Autodesk Inventor part; units mm, degrees
(part 5 of 13)
  line L1582 (2.4, 58.0134) -> (2.4, 59.1669)
  arc A1584 (2.4, 59.1669) -> (2.274, 59.1669) centre (2.337, 59.1669) ccw
  line L1583 (2.274, 59.1669) -> (2.274, 58.0134)
  arc A1585 (2.274, 58.0134) -> (2.4, 58.0134) centre (2.337, 58.0134) ccw
  line L1584 (2.337, 59.2299) -> (2.1578, 59.2299)
  arc A1586 (2.1578, 59.2299) -> (2.1578, 59.1039) centre (2.1578, 59.1669) ccw
  line L1585 (2.1578, 59.1039) -> (2.337, 59.1039)
  arc A1587 (2.337, 59.1039) -> (2.337, 59.2299) centre (2.337, 59.1669) ccw
  line L1586 (2.1337, 59.2251) -> (1.6865, 59.0398)
  arc A1588 (1.6865, 59.0398) -> (1.7347, 58.9234) centre (1.7106, 58.9816) ccw
  line L1587 (1.7347, 58.9234) -> (2.1819, 59.1087)
  arc A1589 (2.1819, 59.1087) -> (2.1337, 59.2251) centre (2.1578, 59.1669) ccw
  line L1588 (1.6661, 59.0261) -> (1.3238, 58.6838)
  arc A1590 (1.3238, 58.6838) -> (1.4128, 58.5948) centre (1.3683, 58.6393) ccw
  line L1589 (1.4128, 58.5948) -> (1.7551, 58.9371)
  arc A1591 (1.7551, 58.9371) -> (1.6661, 59.0261) centre (1.7106, 58.9816) ccw
  line L1590 (1.3101, 58.6634) -> (1.1248, 58.2162)
  arc A1592 (1.1248, 58.2162) -> (1.2412, 58.168) centre (1.183, 58.1921) ccw
  line L1591 (1.2412, 58.168) -> (1.4265, 58.6152)
  arc A1593 (1.4265, 58.6152) -> (1.3101, 58.6634) centre (1.3683, 58.6393) ccw
  line L1592 (1.12, 58.1921) -> (1.12, 58.0128)
  arc A1594 (1.12, 58.0128) -> (1.246, 58.0128) centre (1.183, 58.0128) ccw
  line L1593 (1.246, 58.0128) -> (1.246, 58.1921)
  arc A1595 (1.246, 58.1921) -> (1.12, 58.1921) centre (1.183, 58.1921) ccw
  line L1594 (1.183, 57.9498) -> (2.3365, 57.9498)
  arc A1596 (2.3365, 57.9498) -> (2.3365, 58.0758) centre (2.3365, 58.0128) ccw
  line L1595 (2.3365, 58.0758) -> (1.183, 58.0758)
  arc A1597 (1.183, 58.0758) -> (1.183, 57.9498) centre (1.183, 58.0128) ccw
  line L1596 (2.2735, 58.0128) -> (2.2735, 57.887)
  arc A1598 (2.2735, 57.887) -> (2.3995, 57.887) centre (2.3365, 57.887) ccw
  line L1597 (2.3995, 57.887) -> (2.3995, 58.0128)
  arc A1599 (2.3995, 58.0128) -> (2.2735, 58.0128) centre (2.3365, 58.0128) ccw
  line L1598 (2.3365, 57.95) -> (1.183, 57.95)
  arc A1600 (1.183, 57.95) -> (1.183, 57.824) centre (1.183, 57.887) ccw
  line L1599 (1.183, 57.824) -> (2.3365, 57.824)
  arc A1601 (2.3365, 57.824) -> (2.3365, 57.95) centre (2.3365, 57.887) ccw
  line L1600 (1.12, 57.887) -> (1.12, 57.7078)
  arc A1602 (1.12, 57.7078) -> (1.246, 57.7078) centre (1.183, 57.7078) ccw
  line L1601 (1.246, 57.7078) -> (1.246, 57.887)
  arc A1603 (1.246, 57.887) -> (1.12, 57.887) centre (1.183, 57.887) ccw
  line L1602 (1.1248, 57.6837) -> (1.3101, 57.2365)
  arc A1604 (1.3101, 57.2365) -> (1.4265, 57.2847) centre (1.3683, 57.2606) ccw
  line L1603 (1.4265, 57.2847) -> (1.2412, 57.7319)
  arc A1605 (1.2412, 57.7319) -> (1.1248, 57.6837) centre (1.183, 57.7078) ccw
  line L1604 (1.3238, 57.2161) -> (1.6661, 56.8738)
  arc A1606 (1.6661, 56.8738) -> (1.7551, 56.9628) centre (1.7106, 56.9183) ccw
  line L1605 (1.7551, 56.9628) -> (1.4128, 57.3051)
  arc A1607 (1.4128, 57.3051) -> (1.3238, 57.2161) centre (1.3683, 57.2606) ccw
  line L1606 (1.6865, 56.8601) -> (2.1337, 56.6748)
  arc A1608 (2.1337, 56.6748) -> (2.1819, 56.7912) centre (2.1578, 56.733) ccw
  line L1607 (2.1819, 56.7912) -> (1.7347, 56.9765)
  arc A1609 (1.7347, 56.9765) -> (1.6865, 56.8601) centre (1.7106, 56.9183) ccw
  line L1608 (3.5783, 54.2281) -> (3.5783, 54.6718)
  arc A1610 (3.5783, 54.6718) -> (3.4523, 54.6718) centre (3.5153, 54.6718) ccw
  line L1609 (3.4523, 54.6718) -> (3.4523, 54.2281)
  arc A1611 (3.4523, 54.2281) -> (3.5783, 54.2281) centre (3.5153, 54.2281) ccw
  line L1610 (3.5735, 54.6959) -> (3.4037, 55.1059)
  arc A1612 (3.4037, 55.1059) -> (3.2873, 55.0577) centre (3.3455, 55.0818) ccw
  line L1611 (3.2873, 55.0577) -> (3.4571, 54.6477)
  arc A1613 (3.4571, 54.6477) -> (3.5735, 54.6959) centre (3.5153, 54.6718) ccw
  line L1612 (3.39, 55.1263) -> (3.0763, 55.44)
  arc A1614 (3.0763, 55.44) -> (2.9873, 55.351) centre (3.0318, 55.3955) ccw
  line L1613 (2.9873, 55.351) -> (3.301, 55.0373)
  arc A1615 (3.301, 55.0373) -> (3.39, 55.1263) centre (3.3455, 55.0818) ccw
  line L1614 (3.0559, 55.4537) -> (2.6459, 55.6235)
  arc A1616 (2.6459, 55.6235) -> (2.5977, 55.5071) centre (2.6218, 55.5653) ccw
  line L1615 (2.5977, 55.5071) -> (3.0077, 55.3373)
  arc A1617 (3.0077, 55.3373) -> (3.0559, 55.4537) centre (3.0318, 55.3955) ccw
  line L1616 (2.6218, 55.6283) -> (2.1781, 55.6283)
  arc A1618 (2.1781, 55.6283) -> (2.1781, 55.5023) centre (2.1781, 55.5653) ccw
  line L1617 (2.1781, 55.5023) -> (2.6218, 55.5023)
  arc A1619 (2.6218, 55.5023) -> (2.6218, 55.6283) centre (2.6218, 55.5653) ccw
  line L1618 (2.154, 55.6235) -> (1.744, 55.4537)
  arc A1620 (1.744, 55.4537) -> (1.7922, 55.3373) centre (1.7681, 55.3955) ccw
  line L1619 (1.7922, 55.3373) -> (2.2022, 55.5071)
  arc A1621 (2.2022, 55.5071) -> (2.154, 55.6235) centre (2.1781, 55.5653) ccw
  line L1620 (1.7236, 55.44) -> (1.4099, 55.1263)
  arc A1622 (1.4099, 55.1263) -> (1.4989, 55.0373) centre (1.4544, 55.0818) ccw
  line L1621 (1.4989, 55.0373) -> (1.8126, 55.351)
  arc A1623 (1.8126, 55.351) -> (1.7236, 55.44) centre (1.7681, 55.3955) ccw
  line L1622 (1.3962, 55.1059) -> (1.2264, 54.6959)
  arc A1624 (1.2264, 54.6959) -> (1.3428, 54.6477) centre (1.2846, 54.6718) ccw
  line L1623 (1.3428, 54.6477) -> (1.5126, 55.0577)
  arc A1625 (1.5126, 55.0577) -> (1.3962, 55.1059) centre (1.4544, 55.0818) ccw
  line L1624 (1.2216, 54.6718) -> (1.2216, 54.2281)
  arc A1626 (1.2216, 54.2281) -> (1.3476, 54.2281) centre (1.2846, 54.2281) ccw
  line L1625 (1.3476, 54.2281) -> (1.3476, 54.6718)
  arc A1627 (1.3476, 54.6718) -> (1.2216, 54.6718) centre (1.2846, 54.6718) ccw
  line L1626 (1.2264, 54.204) -> (1.3962, 53.794)
  arc A1628 (1.3962, 53.794) -> (1.5126, 53.8422) centre (1.4544, 53.8181) ccw
  line L1627 (1.5126, 53.8422) -> (1.3428, 54.2522)
  arc A1629 (1.3428, 54.2522) -> (1.2264, 54.204) centre (1.2846, 54.2281) ccw
  line L1628 (1.4099, 53.7736) -> (1.7236, 53.4599)
  arc A1630 (1.7236, 53.4599) -> (1.8126, 53.5489) centre (1.7681, 53.5044) ccw
  line L1629 (1.8126, 53.5489) -> (1.4989, 53.8626)
  arc A1631 (1.4989, 53.8626) -> (1.4099, 53.7736) centre (1.4544, 53.8181) ccw
  line L1630 (1.744, 53.4462) -> (2.154, 53.2764)
  arc A1632 (2.154, 53.2764) -> (2.2022, 53.3928) centre (2.1781, 53.3346) ccw
  line L1631 (2.2022, 53.3928) -> (1.7922, 53.5626)
  arc A1633 (1.7922, 53.5626) -> (1.744, 53.4462) centre (1.7681, 53.5044) ccw
  line L1632 (2.1781, 53.2716) -> (2.6218, 53.2716)
  arc A1634 (2.6218, 53.2716) -> (2.6218, 53.3976) centre (2.6218, 53.3346) ccw
  line L1633 (2.6218, 53.3976) -> (2.1781, 53.3976)
  arc A1635 (2.1781, 53.3976) -> (2.1781, 53.2716) centre (2.1781, 53.3346) ccw
  line L1634 (2.6459, 53.2764) -> (3.0559, 53.4462)
  arc A1636 (3.0559, 53.4462) -> (3.0077, 53.5626) centre (3.0318, 53.5044) ccw
  line L1635 (3.0077, 53.5626) -> (2.5977, 53.3928)
  arc A1637 (2.5977, 53.3928) -> (2.6459, 53.2764) centre (2.6218, 53.3346) ccw
  line L1636 (3.0763, 53.4599) -> (3.39, 53.7736)
  arc A1638 (3.39, 53.7736) -> (3.301, 53.8626) centre (3.3455, 53.8181) ccw
  line L1637 (3.301, 53.8626) -> (2.9873, 53.5489)
  arc A1639 (2.9873, 53.5489) -> (3.0763, 53.4599) centre (3.0318, 53.5044) ccw
  line L1638 (3.4037, 53.794) -> (3.5735, 54.204)
  arc A1640 (3.5735, 54.204) -> (3.4571, 54.2522) centre (3.5153, 54.2281) ccw
  line L1639 (3.4571, 54.2522) -> (3.2873, 53.8422)
  arc A1641 (3.2873, 53.8422) -> (3.4037, 53.794) centre (3.3455, 53.8181) ccw
  line L1640 (2.1578, 42.67) -> (2.337, 42.67)
  arc A1642 (2.337, 42.67) -> (2.337, 42.796) centre (2.337, 42.733) ccw
  line L1641 (2.337, 42.796) -> (2.1578, 42.796)
  arc A1643 (2.1578, 42.796) -> (2.1578, 42.67) centre (2.1578, 42.733) ccw
  line L1642 (2.4, 42.733) -> (2.4, 43.8865)
  arc A1644 (2.4, 43.8865) -> (2.274, 43.8865) centre (2.337, 43.8865) ccw
  line L1643 (2.274, 43.8865) -> (2.274, 42.733)
  arc A1645 (2.274, 42.733) -> (2.4, 42.733) centre (2.337, 42.733) ccw
  line L1644 (2.337, 43.8235) -> (2.4628, 43.8235)
  arc A1646 (2.4628, 43.8235) -> (2.4628, 43.9495) centre (2.4628, 43.8865) ccw
  line L1645 (2.4628, 43.9495) -> (2.337, 43.9495)
  arc A1647 (2.337, 43.9495) -> (2.337, 43.8235) centre (2.337, 43.8865) ccw
  line L1646 (2.3998, 43.8865) -> (2.3998, 42.733)
  arc A1648 (2.3998, 42.733) -> (2.5258, 42.733) centre (2.4628, 42.733) ccw
  line L1647 (2.5258, 42.733) -> (2.5258, 43.8865)
  arc A1649 (2.5258, 43.8865) -> (2.3998, 43.8865) centre (2.4628, 43.8865) ccw
  line L1648 (2.4628, 42.67) -> (2.6421, 42.67)
  arc A1650 (2.6421, 42.67) -> (2.6421, 42.796) centre (2.6421, 42.733) ccw
  line L1649 (2.6421, 42.796) -> (2.4628, 42.796)
  arc A1651 (2.4628, 42.796) -> (2.4628, 42.67) centre (2.4628, 42.733) ccw
  line L1650 (2.6662, 42.6748) -> (3.1134, 42.8601)
  arc A1652 (3.1134, 42.8601) -> (3.0652, 42.9765) centre (3.0893, 42.9183) ccw
  line L1651 (3.0652, 42.9765) -> (2.618, 42.7912)
  arc A1653 (2.618, 42.7912) -> (2.6662, 42.6748) centre (2.6421, 42.733) ccw
  line L1652 (3.1338, 42.8738) -> (3.4761, 43.2161)
  arc A1654 (3.4761, 43.2161) -> (3.3871, 43.3051) centre (3.4316, 43.2606) ccw
  line L1653 (3.3871, 43.3051) -> (3.0448, 42.9628)
  arc A1655 (3.0448, 42.9628) -> (3.1338, 42.8738) centre (3.0893, 42.9183) ccw
  line L1654 (3.4898, 43.2365) -> (3.6751, 43.6837)
  arc A1656 (3.6751, 43.6837) -> (3.5587, 43.7319) centre (3.6169, 43.7078) ccw
  line L1655 (3.5587, 43.7319) -> (3.3734, 43.2847)
  arc A1657 (3.3734, 43.2847) -> (3.4898, 43.2365) centre (3.4316, 43.2606) ccw
  line L1656 (3.6799, 43.7078) -> (3.6799, 43.887)
  arc A1658 (3.6799, 43.887) -> (3.5539, 43.887) centre (3.6169, 43.887) ccw
  line L1657 (3.5539, 43.887) -> (3.5539, 43.7078)
  arc A1659 (3.5539, 43.7078) -> (3.6799, 43.7078) centre (3.6169, 43.7078) ccw
  line L1658 (3.6169, 43.95) -> (2.4634, 43.95)
  arc A1660 (2.4634, 43.95) -> (2.4634, 43.824) centre (2.4634, 43.887) ccw
  line L1659 (2.4634, 43.824) -> (3.6169, 43.824)
  arc A1661 (3.6169, 43.824) -> (3.6169, 43.95) centre (3.6169, 43.887) ccw
  line L1660 (2.5264, 43.887) -> (2.5264, 44.0128)
  arc A1662 (2.5264, 44.0128) -> (2.4004, 44.0128) centre (2.4634, 44.0128) ccw
  line L1661 (2.4004, 44.0128) -> (2.4004, 43.887)
  arc A1663 (2.4004, 43.887) -> (2.5264, 43.887) centre (2.4634, 43.887) ccw
  line L1662 (2.4634, 43.9498) -> (3.6169, 43.9498)
  arc A1664 (3.6169, 43.9498) -> (3.6169, 44.0758) centre (3.6169, 44.0128) ccw
  line L1663 (3.6169, 44.0758) -> (2.4634, 44.0758)
  arc A1665 (2.4634, 44.0758) -> (2.4634, 43.9498) centre (2.4634, 44.0128) ccw
  line L1664 (3.6799, 44.0128) -> (3.6799, 44.1921)
  arc A1666 (3.6799, 44.1921) -> (3.5539, 44.1921) centre (3.6169, 44.1921) ccw
  line L1665 (3.5539, 44.1921) -> (3.5539, 44.0128)
  arc A1667 (3.5539, 44.0128) -> (3.6799, 44.0128) centre (3.6169, 44.0128) ccw
  line L1666 (3.6751, 44.2162) -> (3.4898, 44.6634)
  arc A1668 (3.4898, 44.6634) -> (3.3734, 44.6152) centre (3.4316, 44.6393) ccw
  line L1667 (3.3734, 44.6152) -> (3.5587, 44.168)
  arc A1669 (3.5587, 44.168) -> (3.6751, 44.2162) centre (3.6169, 44.1921) ccw
  line L1668 (3.4761, 44.6838) -> (3.1338, 45.0261)
  arc A1670 (3.1338, 45.0261) -> (3.0448, 44.9371) centre (3.0893, 44.9816) ccw
  line L1669 (3.0448, 44.9371) -> (3.3871, 44.5948)
  arc A1671 (3.3871, 44.5948) -> (3.4761, 44.6838) centre (3.4316, 44.6393) ccw
  line L1670 (3.1134, 45.0398) -> (2.6662, 45.2251)
  arc A1672 (2.6662, 45.2251) -> (2.618, 45.1087) centre (2.6421, 45.1669) ccw
  line L1671 (2.618, 45.1087) -> (3.0652, 44.9234)
  arc A1673 (3.0652, 44.9234) -> (3.1134, 45.0398) centre (3.0893, 44.9816) ccw
  line L1672 (2.6421, 45.2299) -> (2.4628, 45.2299)
  arc A1674 (2.4628, 45.2299) -> (2.4628, 45.1039) centre (2.4628, 45.1669) ccw
  line L1673 (2.4628, 45.1039) -> (2.6421, 45.1039)
  arc A1675 (2.6421, 45.1039) -> (2.6421, 45.2299) centre (2.6421, 45.1669) ccw
  line L1674 (2.3998, 45.1669) -> (2.3998, 44.0134)
  arc A1676 (2.3998, 44.0134) -> (2.5258, 44.0134) centre (2.4628, 44.0134) ccw
  line L1675 (2.5258, 44.0134) -> (2.5258, 45.1669)
  arc A1677 (2.5258, 45.1669) -> (2.3998, 45.1669) centre (2.4628, 45.1669) ccw
  line L1676 (2.4628, 44.0764) -> (2.337, 44.0764)
  arc A1678 (2.337, 44.0764) -> (2.337, 43.9504) centre (2.337, 44.0134) ccw
  line L1677 (2.337, 43.9504) -> (2.4628, 43.9504)
  arc A1679 (2.4628, 43.9504) -> (2.4628, 44.0764) centre (2.4628, 44.0134) ccw
  line L1678 (2.4, 44.0134) -> (2.4, 45.1669)
  arc A1680 (2.4, 45.1669) -> (2.274, 45.1669) centre (2.337, 45.1669) ccw
  line L1679 (2.274, 45.1669) -> (2.274, 44.0134)
  arc A1681 (2.274, 44.0134) -> (2.4, 44.0134) centre (2.337, 44.0134) ccw
  line L1680 (2.337, 45.2299) -> (2.1578, 45.2299)
  arc A1682 (2.1578, 45.2299) -> (2.1578, 45.1039) centre (2.1578, 45.1669) ccw
  line L1681 (2.1578, 45.1039) -> (2.337, 45.1039)
  arc A1683 (2.337, 45.1039) -> (2.337, 45.2299) centre (2.337, 45.1669) ccw
  line L1682 (2.1337, 45.2251) -> (1.6865, 45.0398)
  arc A1684 (1.6865, 45.0398) -> (1.7347, 44.9234) centre (1.7106, 44.9816) ccw
  line L1683 (1.7347, 44.9234) -> (2.1819, 45.1087)
  arc A1685 (2.1819, 45.1087) -> (2.1337, 45.2251) centre (2.1578, 45.1669) ccw
  line L1684 (1.6661, 45.0261) -> (1.3238, 44.6838)
  arc A1686 (1.3238, 44.6838) -> (1.4128, 44.5948) centre (1.3683, 44.6393) ccw
  line L1685 (1.4128, 44.5948) -> (1.7551, 44.9371)
  arc A1687 (1.7551, 44.9371) -> (1.6661, 45.0261) centre (1.7106, 44.9816) ccw
  line L1686 (1.3101, 44.6634) -> (1.1248, 44.2162)
  arc A1688 (1.1248, 44.2162) -> (1.2412, 44.168) centre (1.183, 44.1921) ccw
  line L1687 (1.2412, 44.168) -> (1.4265, 44.6152)
  arc A1689 (1.4265, 44.6152) -> (1.3101, 44.6634) centre (1.3683, 44.6393) ccw
  line L1688 (1.12, 44.1921) -> (1.12, 44.0128)
  arc A1690 (1.12, 44.0128) -> (1.246, 44.0128) centre (1.183, 44.0128) ccw
  line L1689 (1.246, 44.0128) -> (1.246, 44.1921)
  arc A1691 (1.246, 44.1921) -> (1.12, 44.1921) centre (1.183, 44.1921) ccw
  line L1690 (1.183, 43.9498) -> (2.3365, 43.9498)
  arc A1692 (2.3365, 43.9498) -> (2.3365, 44.0758) centre (2.3365, 44.0128) ccw
  line L1691 (2.3365, 44.0758) -> (1.183, 44.0758)
  arc A1693 (1.183, 44.0758) -> (1.183, 43.9498) centre (1.183, 44.0128) ccw
  line L1692 (2.2735, 44.0128) -> (2.2735, 43.887)
  arc A1694 (2.2735, 43.887) -> (2.3995, 43.887) centre (2.3365, 43.887) ccw
  line L1693 (2.3995, 43.887) -> (2.3995, 44.0128)
  arc A1695 (2.3995, 44.0128) -> (2.2735, 44.0128) centre (2.3365, 44.0128) ccw
  line L1694 (2.3365, 43.95) -> (1.183, 43.95)
  arc A1696 (1.183, 43.95) -> (1.183, 43.824) centre (1.183, 43.887) ccw
  line L1695 (1.183, 43.824) -> (2.3365, 43.824)
  arc A1697 (2.3365, 43.824) -> (2.3365, 43.95) centre (2.3365, 43.887) ccw
  line L1696 (1.12, 43.887) -> (1.12, 43.7078)
  arc A1698 (1.12, 43.7078) -> (1.246, 43.7078) centre (1.183, 43.7078) ccw
  line L1697 (1.246, 43.7078) -> (1.246, 43.887)
  arc A1699 (1.246, 43.887) -> (1.12, 43.887) centre (1.183, 43.887) ccw
  line L1698 (1.1248, 43.6837) -> (1.3101, 43.2365)
  arc A1700 (1.3101, 43.2365) -> (1.4265, 43.2847) centre (1.3683, 43.2606) ccw
  line L1699 (1.4265, 43.2847) -> (1.2412, 43.7319)
  arc A1701 (1.2412, 43.7319) -> (1.1248, 43.6837) centre (1.183, 43.7078) ccw
  line L1700 (1.3238, 43.2161) -> (1.6661, 42.8738)
  arc A1702 (1.6661, 42.8738) -> (1.7551, 42.9628) centre (1.7106, 42.9183) ccw
  line L1701 (1.7551, 42.9628) -> (1.4128, 43.3051)
  arc A1703 (1.4128, 43.3051) -> (1.3238, 43.2161) centre (1.3683, 43.2606) ccw
  line L1702 (1.6865, 42.8601) -> (2.1337, 42.6748)
  arc A1704 (2.1337, 42.6748) -> (2.1819, 42.7912) centre (2.1578, 42.733) ccw
  line L1703 (2.1819, 42.7912) -> (1.7347, 42.9765)
  arc A1705 (1.7347, 42.9765) -> (1.6865, 42.8601) centre (1.7106, 42.9183) ccw
  line L1704 (3.5783, 40.2281) -> (3.5783, 40.6718)
  arc A1706 (3.5783, 40.6718) -> (3.4523, 40.6718) centre (3.5153, 40.6718) ccw
  line L1705 (3.4523, 40.6718) -> (3.4523, 40.2281)
  arc A1707 (3.4523, 40.2281) -> (3.5783, 40.2281) centre (3.5153, 40.2281) ccw
  line L1706 (3.5735, 40.6959) -> (3.4037, 41.1059)
  arc A1708 (3.4037, 41.1059) -> (3.2873, 41.0577) centre (3.3455, 41.0818) ccw
  line L1707 (3.2873, 41.0577) -> (3.4571, 40.6477)
  arc A1709 (3.4571, 40.6477) -> (3.5735, 40.6959) centre (3.5153, 40.6718) ccw
  line L1708 (3.39, 41.1263) -> (3.0763, 41.44)
  arc A1710 (3.0763, 41.44) -> (2.9873, 41.351) centre (3.0318, 41.3955) ccw
  line L1709 (2.9873, 41.351) -> (3.301, 41.0373)
  arc A1711 (3.301, 41.0373) -> (3.39, 41.1263) centre (3.3455, 41.0818) ccw
  line L1710 (3.0559, 41.4537) -> (2.6459, 41.6235)
  arc A1712 (2.6459, 41.6235) -> (2.5977, 41.5071) centre (2.6218, 41.5653) ccw
  line L1711 (2.5977, 41.5071) -> (3.0077, 41.3373)
  arc A1713 (3.0077, 41.3373) -> (3.0559, 41.4537) centre (3.0318, 41.3955) ccw
  line L1712 (2.6218, 41.6283) -> (2.1781, 41.6283)
  arc A1714 (2.1781, 41.6283) -> (2.1781, 41.5023) centre (2.1781, 41.5653) ccw
  line L1713 (2.1781, 41.5023) -> (2.6218, 41.5023)
  arc A1715 (2.6218, 41.5023) -> (2.6218, 41.6283) centre (2.6218, 41.5653) ccw
  line L1714 (2.154, 41.6235) -> (1.744, 41.4537)
  arc A1716 (1.744, 41.4537) -> (1.7922, 41.3373) centre (1.7681, 41.3955) ccw
  line L1715 (1.7922, 41.3373) -> (2.2022, 41.5071)
  arc A1717 (2.2022, 41.5071) -> (2.154, 41.6235) centre (2.1781, 41.5653) ccw
  line L1716 (1.7236, 41.44) -> (1.4099, 41.1263)
  arc A1718 (1.4099, 41.1263) -> (1.4989, 41.0373) centre (1.4544, 41.0818) ccw
  line L1717 (1.4989, 41.0373) -> (1.8126, 41.351)
  arc A1719 (1.8126, 41.351) -> (1.7236, 41.44) centre (1.7681, 41.3955) ccw
  line L1718 (1.3962, 41.1059) -> (1.2264, 40.6959)
  arc A1720 (1.2264, 40.6959) -> (1.3428, 40.6477) centre (1.2846, 40.6718) ccw
  line L1719 (1.3428, 40.6477) -> (1.5126, 41.0577)
  arc A1721 (1.5126, 41.0577) -> (1.3962, 41.1059) centre (1.4544, 41.0818) ccw
  line L1720 (1.2216, 40.6718) -> (1.2216, 40.2281)
  arc A1722 (1.2216, 40.2281) -> (1.3476, 40.2281) centre (1.2846, 40.2281) ccw
  line L1721 (1.3476, 40.2281) -> (1.3476, 40.6718)
  arc A1723 (1.3476, 40.6718) -> (1.2216, 40.6718) centre (1.2846, 40.6718) ccw
  line L1722 (1.2264, 40.204) -> (1.3962, 39.794)
  arc A1724 (1.3962, 39.794) -> (1.5126, 39.8422) centre (1.4544, 39.8181) ccw
  line L1723 (1.5126, 39.8422) -> (1.3428, 40.2522)
  arc A1725 (1.3428, 40.2522) -> (1.2264, 40.204) centre (1.2846, 40.2281) ccw
  line L1724 (1.4099, 39.7736) -> (1.7236, 39.4599)
  arc A1726 (1.7236, 39.4599) -> (1.8126, 39.5489) centre (1.7681, 39.5044) ccw
  line L1725 (1.8126, 39.5489) -> (1.4989, 39.8626)
  arc A1727 (1.4989, 39.8626) -> (1.4099, 39.7736) centre (1.4544, 39.8181) ccw
  line L1726 (1.744, 39.4462) -> (2.154, 39.2764)
  arc A1728 (2.154, 39.2764) -> (2.2022, 39.3928) centre (2.1781, 39.3346) ccw
  line L1727 (2.2022, 39.3928) -> (1.7922, 39.5626)
  arc A1729 (1.7922, 39.5626) -> (1.744, 39.4462) centre (1.7681, 39.5044) ccw
  line L1728 (2.1781, 39.2716) -> (2.6218, 39.2716)
  arc A1730 (2.6218, 39.2716) -> (2.6218, 39.3976) centre (2.6218, 39.3346) ccw
  line L1729 (2.6218, 39.3976) -> (2.1781, 39.3976)
  arc A1731 (2.1781, 39.3976) -> (2.1781, 39.2716) centre (2.1781, 39.3346) ccw
  line L1730 (2.6459, 39.2764) -> (3.0559, 39.4462)
  arc A1732 (3.0559, 39.4462) -> (3.0077, 39.5626) centre (3.0318, 39.5044) ccw
  line L1731 (3.0077, 39.5626) -> (2.5977, 39.3928)
  arc A1733 (2.5977, 39.3928) -> (2.6459, 39.2764) centre (2.6218, 39.3346) ccw
  line L1732 (3.0763, 39.4599) -> (3.39, 39.7736)
  arc A1734 (3.39, 39.7736) -> (3.301, 39.8626) centre (3.3455, 39.8181) ccw
  line L1733 (3.301, 39.8626) -> (2.9873, 39.5489)
  arc A1735 (2.9873, 39.5489) -> (3.0763, 39.4599) centre (3.0318, 39.5044) ccw
  line L1734 (3.4037, 39.794) -> (3.5735, 40.204)
  arc A1736 (3.5735, 40.204) -> (3.4571, 40.2522) centre (3.5153, 40.2281) ccw
  line L1735 (3.4571, 40.2522) -> (3.2873, 39.8422)
  arc A1737 (3.2873, 39.8422) -> (3.4037, 39.794) centre (3.3455, 39.8181) ccw
  line L1736 (2.1578, 28.67) -> (2.337, 28.67)
  arc A1738 (2.337, 28.67) -> (2.337, 28.796) centre (2.337, 28.733) ccw
  line L1737 (2.337, 28.796) -> (2.1578, 28.796)
  arc A1739 (2.1578, 28.796) -> (2.1578, 28.67) centre (2.1578, 28.733) ccw
  line L1738 (2.4, 28.733) -> (2.4, 29.8865)
  arc A1740 (2.4, 29.8865) -> (2.274, 29.8865) centre (2.337, 29.8865) ccw
  line L1739 (2.274, 29.8865) -> (2.274, 28.733)
  arc A1741 (2.274, 28.733) -> (2.4, 28.733) centre (2.337, 28.733) ccw
  line L1740 (2.337, 29.8235) -> (2.4628, 29.8235)
  arc A1742 (2.4628, 29.8235) -> (2.4628, 29.9495) centre (2.4628, 29.8865) ccw
  line L1741 (2.4628, 29.9495) -> (2.337, 29.9495)
  arc A1743 (2.337, 29.9495) -> (2.337, 29.8235) centre (2.337, 29.8865) ccw
  line L1742 (2.3998, 29.8865) -> (2.3998, 28.733)
  arc A1744 (2.3998, 28.733) -> (2.5258, 28.733) centre (2.4628, 28.733) ccw
  line L1743 (2.5258, 28.733) -> (2.5258, 29.8865)
  arc A1745 (2.5258, 29.8865) -> (2.3998, 29.8865) centre (2.4628, 29.8865) ccw
  line L1744 (2.4628, 28.67) -> (2.6421, 28.67)
  arc A1746 (2.6421, 28.67) -> (2.6421, 28.796) centre (2.6421, 28.733) ccw
  line L1745 (2.6421, 28.796) -> (2.4628, 28.796)
  arc A1747 (2.4628, 28.796) -> (2.4628, 28.67) centre (2.4628, 28.733) ccw
  line L1746 (2.6662, 28.6748) -> (3.1134, 28.8601)
  arc A1748 (3.1134, 28.8601) -> (3.0652, 28.9765) centre (3.0893, 28.9183) ccw
  line L1747 (3.0652, 28.9765) -> (2.618, 28.7912)
  arc A1749 (2.618, 28.7912) -> (2.6662, 28.6748) centre (2.6421, 28.733) ccw
  line L1748 (3.1338, 28.8738) -> (3.4761, 29.2161)
  arc A1750 (3.4761, 29.2161) -> (3.3871, 29.3051) centre (3.4316, 29.2606) ccw
  line L1749 (3.3871, 29.3051) -> (3.0448, 28.9628)
  arc A1751 (3.0448, 28.9628) -> (3.1338, 28.8738) centre (3.0893, 28.9183) ccw
  line L1750 (3.4898, 29.2365) -> (3.6751, 29.6837)
  arc A1752 (3.6751, 29.6837) -> (3.5587, 29.7319) centre (3.6169, 29.7078) ccw
  line L1751 (3.5587, 29.7319) -> (3.3734, 29.2847)
  arc A1753 (3.3734, 29.2847) -> (3.4898, 29.2365) centre (3.4316, 29.2606) ccw
  line L1752 (3.6799, 29.7078) -> (3.6799, 29.887)
  arc A1754 (3.6799, 29.887) -> (3.5539, 29.887) centre (3.6169, 29.887) ccw
  line L1753 (3.5539, 29.887) -> (3.5539, 29.7078)
  arc A1755 (3.5539, 29.7078) -> (3.6799, 29.7078) centre (3.6169, 29.7078) ccw
  line L1754 (3.6169, 29.95) -> (2.4634, 29.95)
  arc A1756 (2.4634, 29.95) -> (2.4634, 29.824) centre (2.4634, 29.887) ccw
  line L1755 (2.4634, 29.824) -> (3.6169, 29.824)
  arc A1757 (3.6169, 29.824) -> (3.6169, 29.95) centre (3.6169, 29.887) ccw
  line L1756 (2.5264, 29.887) -> (2.5264, 30.0128)
  arc A1758 (2.5264, 30.0128) -> (2.4004, 30.0128) centre (2.4634, 30.0128) ccw
  line L1757 (2.4004, 30.0128) -> (2.4004, 29.887)
  arc A1759 (2.4004, 29.887) -> (2.5264, 29.887) centre (2.4634, 29.887) ccw
  line L1758 (2.4634, 29.9498) -> (3.6169, 29.9498)
  arc A1760 (3.6169, 29.9498) -> (3.6169, 30.0758) centre (3.6169, 30.0128) ccw
  line L1759 (3.6169, 30.0758) -> (2.4634, 30.0758)
  arc A1761 (2.4634, 30.0758) -> (2.4634, 29.9498) centre (2.4634, 30.0128) ccw
  line L1760 (3.6799, 30.0128) -> (3.6799, 30.1921)
  arc A1762 (3.6799, 30.1921) -> (3.5539, 30.1921) centre (3.6169, 30.1921) ccw
  line L1761 (3.5539, 30.1921) -> (3.5539, 30.0128)
  arc A1763 (3.5539, 30.0128) -> (3.6799, 30.0128) centre (3.6169, 30.0128) ccw
  line L1762 (3.6751, 30.2162) -> (3.4898, 30.6634)
  arc A1764 (3.4898, 30.6634) -> (3.3734, 30.6152) centre (3.4316, 30.6393) ccw
  line L1763 (3.3734, 30.6152) -> (3.5587, 30.168)
  arc A1765 (3.5587, 30.168) -> (3.6751, 30.2162) centre (3.6169, 30.1921) ccw
  line L1764 (3.4761, 30.6838) -> (3.1338, 31.0261)
  arc A1766 (3.1338, 31.0261) -> (3.0448, 30.9371) centre (3.0893, 30.9816) ccw
  line L1765 (3.0448, 30.9371) -> (3.3871, 30.5948)
  arc A1767 (3.3871, 30.5948) -> (3.4761, 30.6838) centre (3.4316, 30.6393) ccw
  line L1766 (3.1134, 31.0398) -> (2.6662, 31.2251)
  arc A1768 (2.6662, 31.2251) -> (2.618, 31.1087) centre (2.6421, 31.1669) ccw
  line L1767 (2.618, 31.1087) -> (3.0652, 30.9234)
  arc A1769 (3.0652, 30.9234) -> (3.1134, 31.0398) centre (3.0893, 30.9816) ccw
  line L1768 (2.6421, 31.2299) -> (2.4628, 31.2299)
  arc A1770 (2.4628, 31.2299) -> (2.4628, 31.1039) centre (2.4628, 31.1669) ccw
  line L1769 (2.4628, 31.1039) -> (2.6421, 31.1039)
  arc A1771 (2.6421, 31.1039) -> (2.6421, 31.2299) centre (2.6421, 31.1669) ccw
  line L1770 (2.3998, 31.1669) -> (2.3998, 30.0134)
  arc A1772 (2.3998, 30.0134) -> (2.5258, 30.0134) centre (2.4628, 30.0134) ccw
  line L1771 (2.5258, 30.0134) -> (2.5258, 31.1669)
  arc A1773 (2.5258, 31.1669) -> (2.3998, 31.1669) centre (2.4628, 31.1669) ccw
  line L1772 (2.4628, 30.0764) -> (2.337, 30.0764)
  arc A1774 (2.337, 30.0764) -> (2.337, 29.9504) centre (2.337, 30.0134) ccw
  line L1773 (2.337, 29.9504) -> (2.4628, 29.9504)
  arc A1775 (2.4628, 29.9504) -> (2.4628, 30.0764) centre (2.4628, 30.0134) ccw
  line L1774 (2.4, 30.0134) -> (2.4, 31.1669)
  arc A1776 (2.4, 31.1669) -> (2.274, 31.1669) centre (2.337, 31.1669) ccw
  line L1775 (2.274, 31.1669) -> (2.274, 30.0134)
  arc A1777 (2.274, 30.0134) -> (2.4, 30.0134) centre (2.337, 30.0134) ccw
  line L1776 (2.337, 31.2299) -> (2.1578, 31.2299)
  arc A1778 (2.1578, 31.2299) -> (2.1578, 31.1039) centre (2.1578, 31.1669) ccw
  line L1777 (2.1578, 31.1039) -> (2.337, 31.1039)
  arc A1779 (2.337, 31.1039) -> (2.337, 31.2299) centre (2.337, 31.1669) ccw
  line L1778 (2.1337, 31.2251) -> (1.6865, 31.0398)
  arc A1780 (1.6865, 31.0398) -> (1.7347, 30.9234) centre (1.7106, 30.9816) ccw
  line L1779 (1.7347, 30.9234) -> (2.1819, 31.1087)
  arc A1781 (2.1819, 31.1087) -> (2.1337, 31.2251) centre (2.1578, 31.1669) ccw
  line L1780 (1.6661, 31.0261) -> (1.3238, 30.6838)
  arc A1782 (1.3238, 30.6838) -> (1.4128, 30.5948) centre (1.3683, 30.6393) ccw
  line L1781 (1.4128, 30.5948) -> (1.7551, 30.9371)
  arc A1783 (1.7551, 30.9371) -> (1.6661, 31.0261) centre (1.7106, 30.9816) ccw
  line L1782 (1.3101, 30.6634) -> (1.1248, 30.2162)
  arc A1784 (1.1248, 30.2162) -> (1.2412, 30.168) centre (1.183, 30.1921) ccw
  line L1783 (1.2412, 30.168) -> (1.4265, 30.6152)
  arc A1785 (1.4265, 30.6152) -> (1.3101, 30.6634) centre (1.3683, 30.6393) ccw
  line L1784 (1.12, 30.1921) -> (1.12, 30.0128)
  arc A1786 (1.12, 30.0128) -> (1.246, 30.0128) centre (1.183, 30.0128) ccw
  line L1785 (1.246, 30.0128) -> (1.246, 30.1921)
  arc A1787 (1.246, 30.1921) -> (1.12, 30.1921) centre (1.183, 30.1921) ccw
  line L1786 (1.183, 29.9498) -> (2.3365, 29.9498)
  arc A1788 (2.3365, 29.9498) -> (2.3365, 30.0758) centre (2.3365, 30.0128) ccw
  line L1787 (2.3365, 30.0758) -> (1.183, 30.0758)
  arc A1789 (1.183, 30.0758) -> (1.183, 29.9498) centre (1.183, 30.0128) ccw
  line L1788 (2.2735, 30.0128) -> (2.2735, 29.887)
  arc A1790 (2.2735, 29.887) -> (2.3995, 29.887) centre (2.3365, 29.887) ccw
  line L1789 (2.3995, 29.887) -> (2.3995, 30.0128)
  arc A1791 (2.3995, 30.0128) -> (2.2735, 30.0128) centre (2.3365, 30.0128) ccw
  line L1790 (2.3365, 29.95) -> (1.183, 29.95)
  arc A1792 (1.183, 29.95) -> (1.183, 29.824) centre (1.183, 29.887) ccw
  line L1791 (1.183, 29.824) -> (2.3365, 29.824)
  arc A1793 (2.3365, 29.824) -> (2.3365, 29.95) centre (2.3365, 29.887) ccw
  line L1792 (1.12, 29.887) -> (1.12, 29.7078)
  arc A1794 (1.12, 29.7078) -> (1.246, 29.7078) centre (1.183, 29.7078) ccw
  line L1793 (1.246, 29.7078) -> (1.246, 29.887)
  arc A1795 (1.246, 29.887) -> (1.12, 29.887) centre (1.183, 29.887) ccw
  line L1794 (1.1248, 29.6837) -> (1.3101, 29.2365)
  arc A1796 (1.3101, 29.2365) -> (1.4265, 29.2847) centre (1.3683, 29.2606) ccw
  line L1795 (1.4265, 29.2847) -> (1.2412, 29.7319)
  arc A1797 (1.2412, 29.7319) -> (1.1248, 29.6837) centre (1.183, 29.7078) ccw
  line L1796 (1.3238, 29.2161) -> (1.6661, 28.8738)
  arc A1798 (1.6661, 28.8738) -> (1.7551, 28.9628) centre (1.7106, 28.9183) ccw
  line L1797 (1.7551, 28.9628) -> (1.4128, 29.3051)
  arc A1799 (1.4128, 29.3051) -> (1.3238, 29.2161) centre (1.3683, 29.2606) ccw
  line L1798 (1.6865, 28.8601) -> (2.1337, 28.6748)
  arc A1800 (2.1337, 28.6748) -> (2.1819, 28.7912) centre (2.1578, 28.733) ccw
  line L1799 (2.1819, 28.7912) -> (1.7347, 28.9765)
  arc A1801 (1.7347, 28.9765) -> (1.6865, 28.8601) centre (1.7106, 28.9183) ccw
  line L1800 (3.5783, 26.2281) -> (3.5783, 26.6718)
  arc A1802 (3.5783, 26.6718) -> (3.4523, 26.6718) centre (3.5153, 26.6718) ccw
  line L1801 (3.4523, 26.6718) -> (3.4523, 26.2281)
  arc A1803 (3.4523, 26.2281) -> (3.5783, 26.2281) centre (3.5153, 26.2281) ccw
  line L1802 (3.5735, 26.6959) -> (3.4037, 27.1059)
  arc A1804 (3.4037, 27.1059) -> (3.2873, 27.0577) centre (3.3455, 27.0818) ccw
  line L1803 (3.2873, 27.0577) -> (3.4571, 26.6477)
  arc A1805 (3.4571, 26.6477) -> (3.5735, 26.6959) centre (3.5153, 26.6718) ccw
  line L1804 (3.39, 27.1263) -> (3.0763, 27.44)
  arc A1806 (3.0763, 27.44) -> (2.9873, 27.351) centre (3.0318, 27.3955) ccw
  line L1805 (2.9873, 27.351) -> (3.301, 27.0373)
  arc A1807 (3.301, 27.0373) -> (3.39, 27.1263) centre (3.3455, 27.0818) ccw
  line L1806 (3.0559, 27.4537) -> (2.6459, 27.6235)
  arc A1808 (2.6459, 27.6235) -> (2.5977, 27.5071) centre (2.6218, 27.5653) ccw
  line L1807 (2.5977, 27.5071) -> (3.0077, 27.3373)
  arc A1809 (3.0077, 27.3373) -> (3.0559, 27.4537) centre (3.0318, 27.3955) ccw
  line L1808 (2.6218, 27.6283) -> (2.1781, 27.6283)
  arc A1810 (2.1781, 27.6283) -> (2.1781, 27.5023) centre (2.1781, 27.5653) ccw
  line L1809 (2.1781, 27.5023) -> (2.6218, 27.5023)
  arc A1811 (2.6218, 27.5023) -> (2.6218, 27.6283) centre (2.6218, 27.5653) ccw
  line L1810 (2.154, 27.6235) -> (1.744, 27.4537)
  arc A1812 (1.744, 27.4537) -> (1.7922, 27.3373) centre (1.7681, 27.3955) ccw
  line L1811 (1.7922, 27.3373) -> (2.2022, 27.5071)
  arc A1813 (2.2022, 27.5071) -> (2.154, 27.6235) centre (2.1781, 27.5653) ccw
  line L1812 (1.7236, 27.44) -> (1.4099, 27.1263)
  arc A1814 (1.4099, 27.1263) -> (1.4989, 27.0373) centre (1.4544, 27.0818) ccw
  line L1813 (1.4989, 27.0373) -> (1.8126, 27.351)
  arc A1815 (1.8126, 27.351) -> (1.7236, 27.44) centre (1.7681, 27.3955) ccw
  line L1814 (1.3962, 27.1059) -> (1.2264, 26.6959)
  arc A1816 (1.2264, 26.6959) -> (1.3428, 26.6477) centre (1.2846, 26.6718) ccw
  line L1815 (1.3428, 26.6477) -> (1.5126, 27.0577)
  arc A1817 (1.5126, 27.0577) -> (1.3962, 27.1059) centre (1.4544, 27.0818) ccw
  line L1816 (1.2216, 26.6718) -> (1.2216, 26.2281)
  arc A1818 (1.2216, 26.2281) -> (1.3476, 26.2281) centre (1.2846, 26.2281) ccw
  line L1817 (1.3476, 26.2281) -> (1.3476, 26.6718)
  arc A1819 (1.3476, 26.6718) -> (1.2216, 26.6718) centre (1.2846, 26.6718) ccw
  line L1818 (1.2264, 26.204) -> (1.3962, 25.794)
  arc A1820 (1.3962, 25.794) -> (1.5126, 25.8422) centre (1.4544, 25.8181) ccw
  line L1819 (1.5126, 25.8422) -> (1.3428, 26.2522)
  arc A1821 (1.3428, 26.2522) -> (1.2264, 26.204) centre (1.2846, 26.2281) ccw
  line L1820 (1.4099, 25.7736) -> (1.7236, 25.4599)
  arc A1822 (1.7236, 25.4599) -> (1.8126, 25.5489) centre (1.7681, 25.5044) ccw
  line L1821 (1.8126, 25.5489) -> (1.4989, 25.8626)
  arc A1823 (1.4989, 25.8626) -> (1.4099, 25.7736) centre (1.4544, 25.8181) ccw
  line L1822 (1.744, 25.4462) -> (2.154, 25.2764)
  arc A1824 (2.154, 25.2764) -> (2.2022, 25.3928) centre (2.1781, 25.3346) ccw
  line L1823 (2.2022, 25.3928) -> (1.7922, 25.5626)
  arc A1825 (1.7922, 25.5626) -> (1.744, 25.4462) centre (1.7681, 25.5044) ccw
  line L1824 (2.1781, 25.2716) -> (2.6218, 25.2716)
  arc A1826 (2.6218, 25.2716) -> (2.6218, 25.3976) centre (2.6218, 25.3346) ccw
  line L1825 (2.6218, 25.3976) -> (2.1781, 25.3976)
  arc A1827 (2.1781, 25.3976) -> (2.1781, 25.2716) centre (2.1781, 25.3346) ccw
  line L1826 (2.6459, 25.2764) -> (3.0559, 25.4462)
  arc A1828 (3.0559, 25.4462) -> (3.0077, 25.5626) centre (3.0318, 25.5044) ccw
  line L1827 (3.0077, 25.5626) -> (2.5977, 25.3928)
  arc A1829 (2.5977, 25.3928) -> (2.6459, 25.2764) centre (2.6218, 25.3346) ccw
  line L1828 (3.0763, 25.4599) -> (3.39, 25.7736)
  arc A1830 (3.39, 25.7736) -> (3.301, 25.8626) centre (3.3455, 25.8181) ccw
  line L1829 (3.301, 25.8626) -> (2.9873, 25.5489)
  arc A1831 (2.9873, 25.5489) -> (3.0763, 25.4599) centre (3.0318, 25.5044) ccw
  line L1830 (3.4037, 25.794) -> (3.5735, 26.204)
  arc A1832 (3.5735, 26.204) -> (3.4571, 26.2522) centre (3.5153, 26.2281) ccw
  line L1831 (3.4571, 26.2522) -> (3.2873, 25.8422)
  arc A1833 (3.2873, 25.8422) -> (3.4037, 25.794) centre (3.3455, 25.8181) ccw
  line L1832 (3.3892, 20.6283) -> (1.4107, 20.6283)
  arc A1834 (1.4107, 20.6283) -> (1.4107, 20.5023) centre (1.4107, 20.5653) ccw
  line L1833 (1.4107, 20.5023) -> (3.3892, 20.5023)
  arc A1835 (3.3892, 20.5023) -> (3.3892, 20.6283) centre (3.3892, 20.5653) ccw
  line L1834 (1.3662, 20.6098) -> (1.2401, 20.4837)
  arc A1836 (1.2401, 20.4837) -> (1.3291, 20.3947) centre (1.2846, 20.4392) ccw
  line L1835 (1.3291, 20.3947) -> (1.4552, 20.5208)
  arc A1837 (1.4552, 20.5208) -> (1.3662, 20.6098) centre (1.4107, 20.5653) ccw
  line L1836 (1.2216, 20.4392) -> (1.2216, 18.4607)
  arc A1838 (1.2216, 18.4607) -> (1.3476, 18.4607) centre (1.2846, 18.4607) ccw
  line L1837 (1.3476, 18.4607) -> (1.3476, 20.4392)
  arc A1839 (1.3476, 20.4392) -> (1.2216, 20.4392) centre (1.2846, 20.4392) ccw
  line L1838 (1.2401, 18.4162) -> (1.3662, 18.2901)
  arc A1840 (1.3662, 18.2901) -> (1.4552, 18.3791) centre (1.4107, 18.3346) ccw
  line L1839 (1.4552, 18.3791) -> (1.3291, 18.5052)
  arc A1841 (1.3291, 18.5052) -> (1.2401, 18.4162) centre (1.2846, 18.4607) ccw
  line L1840 (1.4107, 18.2716) -> (3.3892, 18.2716)
  arc A1842 (3.3892, 18.2716) -> (3.3892, 18.3976) centre (3.3892, 18.3346) ccw
  line L1841 (3.3892, 18.3976) -> (1.4107, 18.3976)
  arc A1843 (1.4107, 18.3976) -> (1.4107, 18.2716) centre (1.4107, 18.3346) ccw
  line L1842 (3.4337, 18.2901) -> (3.5598, 18.4162)
  arc A1844 (3.5598, 18.4162) -> (3.4708, 18.5052) centre (3.5153, 18.4607) ccw
  line L1843 (3.4708, 18.5052) -> (3.3447, 18.3791)
  arc A1845 (3.3447, 18.3791) -> (3.4337, 18.2901) centre (3.3892, 18.3346) ccw
  line L1844 (3.5783, 18.4607) -> (3.5783, 20.4392)
  arc A1846 (3.5783, 20.4392) -> (3.4523, 20.4392) centre (3.5153, 20.4392) ccw
  line L1845 (3.4523, 20.4392) -> (3.4523, 18.4607)
  arc A1847 (3.4523, 18.4607) -> (3.5783, 18.4607) centre (3.5153, 18.4607) ccw
  line L1846 (3.5598, 20.4837) -> (3.4337, 20.6098)
  arc A1848 (3.4337, 20.6098) -> (3.3447, 20.5208) centre (3.3892, 20.5653) ccw
  line L1847 (3.3447, 20.5208) -> (3.4708, 20.3947)
  arc A1849 (3.4708, 20.3947) -> (3.5598, 20.4837) centre (3.5153, 20.4392) ccw
  line L1848 (2.1578, 21.67) -> (2.337, 21.67)
  arc A1850 (2.337, 21.67) -> (2.337, 21.796) centre (2.337, 21.733) ccw
  line L1849 (2.337, 21.796) -> (2.1578, 21.796)
  arc A1851 (2.1578, 21.796) -> (2.1578, 21.67) centre (2.1578, 21.733) ccw
  line L1850 (2.4, 21.733) -> (2.4, 22.8865)
  arc A1852 (2.4, 22.8865) -> (2.274, 22.8865) centre (2.337, 22.8865) ccw
  line L1851 (2.274, 22.8865) -> (2.274, 21.733)
  arc A1853 (2.274, 21.733) -> (2.4, 21.733) centre (2.337, 21.733) ccw
  line L1852 (2.337, 22.8235) -> (2.4628, 22.8235)
  arc A1854 (2.4628, 22.8235) -> (2.4628, 22.9495) centre (2.4628, 22.8865) ccw
  line L1853 (2.4628, 22.9495) -> (2.337, 22.9495)
  arc A1855 (2.337, 22.9495) -> (2.337, 22.8235) centre (2.337, 22.8865) ccw
  line L1854 (2.3998, 22.8865) -> (2.3998, 21.733)
  arc A1856 (2.3998, 21.733) -> (2.5258, 21.733) centre (2.4628, 21.733) ccw
  line L1855 (2.5258, 21.733) -> (2.5258, 22.8865)
  arc A1857 (2.5258, 22.8865) -> (2.3998, 22.8865) centre (2.4628, 22.8865) ccw
  line L1856 (2.4628, 21.67) -> (2.6421, 21.67)
  arc A1858 (2.6421, 21.67) -> (2.6421, 21.796) centre (2.6421, 21.733) ccw
  line L1857 (2.6421, 21.796) -> (2.4628, 21.796)
  arc A1859 (2.4628, 21.796) -> (2.4628, 21.67) centre (2.4628, 21.733) ccw
  line L1858 (2.6662, 21.6748) -> (3.1134, 21.8601)
  arc A1860 (3.1134, 21.8601) -> (3.0652, 21.9765) centre (3.0893, 21.9183) ccw
  line L1859 (3.0652, 21.9765) -> (2.618, 21.7912)
  arc A1861 (2.618, 21.7912) -> (2.6662, 21.6748) centre (2.6421, 21.733) ccw
  line L1860 (3.1338, 21.8738) -> (3.4761, 22.2161)
  arc A1862 (3.4761, 22.2161) -> (3.3871, 22.3051) centre (3.4316, 22.2606) ccw
  line L1861 (3.3871, 22.3051) -> (3.0448, 21.9628)
  arc A1863 (3.0448, 21.9628) -> (3.1338, 21.8738) centre (3.0893, 21.9183) ccw
  line L1862 (3.4898, 22.2365) -> (3.6751, 22.6837)
  arc A1864 (3.6751, 22.6837) -> (3.5587, 22.7319) centre (3.6169, 22.7078) ccw
  line L1863 (3.5587, 22.7319) -> (3.3734, 22.2847)
  arc A1865 (3.3734, 22.2847) -> (3.4898, 22.2365) centre (3.4316, 22.2606) ccw
  line L1864 (3.6799, 22.7078) -> (3.6799, 22.887)
  arc A1866 (3.6799, 22.887) -> (3.5539, 22.887) centre (3.6169, 22.887) ccw
  line L1865 (3.5539, 22.887) -> (3.5539, 22.7078)
  arc A1867 (3.5539, 22.7078) -> (3.6799, 22.7078) centre (3.6169, 22.7078) ccw
  line L1866 (3.6169, 22.95) -> (2.4634, 22.95)
  arc A1868 (2.4634, 22.95) -> (2.4634, 22.824) centre (2.4634, 22.887) ccw
  line L1867 (2.4634, 22.824) -> (3.6169, 22.824)
  arc A1869 (3.6169, 22.824) -> (3.6169, 22.95) centre (3.6169, 22.887) ccw
  line L1868 (2.5264, 22.887) -> (2.5264, 23.0128)
  arc A1870 (2.5264, 23.0128) -> (2.4004, 23.0128) centre (2.4634, 23.0128) ccw
  line L1869 (2.4004, 23.0128) -> (2.4004, 22.887)
  arc A1871 (2.4004, 22.887) -> (2.5264, 22.887) centre (2.4634, 22.887) ccw
  line L1870 (2.4634, 22.9498) -> (3.6169, 22.9498)
  arc A1872 (3.6169, 22.9498) -> (3.6169, 23.0758) centre (3.6169, 23.0128) ccw
  line L1871 (3.6169, 23.0758) -> (2.4634, 23.0758)
  arc A1873 (2.4634, 23.0758) -> (2.4634, 22.9498) centre (2.4634, 23.0128) ccw
  line L1872 (3.6799, 23.0128) -> (3.6799, 23.1921)
  arc A1874 (3.6799, 23.1921) -> (3.5539, 23.1921) centre (3.6169, 23.1921) ccw
  line L1873 (3.5539, 23.1921) -> (3.5539, 23.0128)
  arc A1875 (3.5539, 23.0128) -> (3.6799, 23.0128) centre (3.6169, 23.0128) ccw
  line L1874 (3.6751, 23.2162) -> (3.4898, 23.6634)
  arc A1876 (3.4898, 23.6634) -> (3.3734, 23.6152) centre (3.4316, 23.6393) ccw
  line L1875 (3.3734, 23.6152) -> (3.5587, 23.168)
  arc A1877 (3.5587, 23.168) -> (3.6751, 23.2162) centre (3.6169, 23.1921) ccw
  line L1876 (3.4761, 23.6838) -> (3.1338, 24.0261)
  arc A1878 (3.1338, 24.0261) -> (3.0448, 23.9371) centre (3.0893, 23.9816) ccw
  line L1877 (3.0448, 23.9371) -> (3.3871, 23.5948)
  arc A1879 (3.3871, 23.5948) -> (3.4761, 23.6838) centre (3.4316, 23.6393) ccw
  line L1878 (3.1134, 24.0398) -> (2.6662, 24.2251)
  arc A1880 (2.6662, 24.2251) -> (2.618, 24.1087) centre (2.6421, 24.1669) ccw
  line L1879 (2.618, 24.1087) -> (3.0652, 23.9234)
  arc A1881 (3.0652, 23.9234) -> (3.1134, 24.0398) centre (3.0893, 23.9816) ccw
  line L1880 (2.6421, 24.2299) -> (2.4628, 24.2299)
  arc A1882 (2.4628, 24.2299) -> (2.4628, 24.1039) centre (2.4628, 24.1669) ccw
  line L1881 (2.4628, 24.1039) -> (2.6421, 24.1039)
  arc A1883 (2.6421, 24.1039) -> (2.6421, 24.2299) centre (2.6421, 24.1669) ccw
  line L1882 (2.3998, 24.1669) -> (2.3998, 23.0134)
  arc A1884 (2.3998, 23.0134) -> (2.5258, 23.0134) centre (2.4628, 23.0134) ccw
  line L1883 (2.5258, 23.0134) -> (2.5258, 24.1669)
  arc A1885 (2.5258, 24.1669) -> (2.3998, 24.1669) centre (2.4628, 24.1669) ccw
  line L1884 (2.4628, 23.0764) -> (2.337, 23.0764)
  arc A1886 (2.337, 23.0764) -> (2.337, 22.9504) centre (2.337, 23.0134) ccw
  line L1885 (2.337, 22.9504) -> (2.4628, 22.9504)
  arc A1887 (2.4628, 22.9504) -> (2.4628, 23.0764) centre (2.4628, 23.0134) ccw
  line L1886 (2.4, 23.0134) -> (2.4, 24.1669)
  arc A1888 (2.4, 24.1669) -> (2.274, 24.1669) centre (2.337, 24.1669) ccw
  line L1887 (2.274, 24.1669) -> (2.274, 23.0134)
  arc A1889 (2.274, 23.0134) -> (2.4, 23.0134) centre (2.337, 23.0134) ccw
  line L1888 (2.337, 24.2299) -> (2.1578, 24.2299)
  arc A1890 (2.1578, 24.2299) -> (2.1578, 24.1039) centre (2.1578, 24.1669) ccw
  line L1889 (2.1578, 24.1039) -> (2.337, 24.1039)
  arc A1891 (2.337, 24.1039) -> (2.337, 24.2299) centre (2.337, 24.1669) ccw
  line L1890 (2.1337, 24.2251) -> (1.6865, 24.0398)
  arc A1892 (1.6865, 24.0398) -> (1.7347, 23.9234) centre (1.7106, 23.9816) ccw
  line L1891 (1.7347, 23.9234) -> (2.1819, 24.1087)
  arc A1893 (2.1819, 24.1087) -> (2.1337, 24.2251) centre (2.1578, 24.1669) ccw
  line L1892 (1.6661, 24.0261) -> (1.3238, 23.6838)
  arc A1894 (1.3238, 23.6838) -> (1.4128, 23.5948) centre (1.3683, 23.6393) ccw
  line L1893 (1.4128, 23.5948) -> (1.7551, 23.9371)
  arc A1895 (1.7551, 23.9371) -> (1.6661, 24.0261) centre (1.7106, 23.9816) ccw
  line L1894 (1.3101, 23.6634) -> (1.1248, 23.2162)
  arc A1896 (1.1248, 23.2162) -> (1.2412, 23.168) centre (1.183, 23.1921) ccw
  line L1895 (1.2412, 23.168) -> (1.4265, 23.6152)
  arc A1897 (1.4265, 23.6152) -> (1.3101, 23.6634) centre (1.3683, 23.6393) ccw
  line L1896 (1.12, 23.1921) -> (1.12, 23.0128)
  arc A1898 (1.12, 23.0128) -> (1.246, 23.0128) centre (1.183, 23.0128) ccw
  line L1897 (1.246, 23.0128) -> (1.246, 23.1921)
  arc A1899 (1.246, 23.1921) -> (1.12, 23.1921) centre (1.183, 23.1921) ccw
  line L1898 (1.183, 22.9498) -> (2.3365, 22.9498)
  arc A1900 (2.3365, 22.9498) -> (2.3365, 23.0758) centre (2.3365, 23.0128) ccw
  line L1899 (2.3365, 23.0758) -> (1.183, 23.0758)
  arc A1901 (1.183, 23.0758) -> (1.183, 22.9498) centre (1.183, 23.0128) ccw
  line L1900 (2.2735, 23.0128) -> (2.2735, 22.887)
  arc A1902 (2.2735, 22.887) -> (2.3995, 22.887) centre (2.3365, 22.887) ccw
  line L1901 (2.3995, 22.887) -> (2.3995, 23.0128)
  arc A1903 (2.3995, 23.0128) -> (2.2735, 23.0128) centre (2.3365, 23.0128) ccw
  line L1902 (2.3365, 22.95) -> (1.183, 22.95)
  arc A1904 (1.183, 22.95) -> (1.183, 22.824) centre (1.183, 22.887) ccw
  line L1903 (1.183, 22.824) -> (2.3365, 22.824)
  arc A1905 (2.3365, 22.824) -> (2.3365, 22.95) centre (2.3365, 22.887) ccw
  line L1904 (1.12, 22.887) -> (1.12, 22.7078)
  arc A1906 (1.12, 22.7078) -> (1.246, 22.7078) centre (1.183, 22.7078) ccw
  line L1905 (1.246, 22.7078) -> (1.246, 22.887)
  arc A1907 (1.246, 22.887) -> (1.12, 22.887) centre (1.183, 22.887) ccw
  line L1906 (1.1248, 22.6837) -> (1.3101, 22.2365)
  arc A1908 (1.3101, 22.2365) -> (1.4265, 22.2847) centre (1.3683, 22.2606) ccw
  line L1907 (1.4265, 22.2847) -> (1.2412, 22.7319)
  arc A1909 (1.2412, 22.7319) -> (1.1248, 22.6837) centre (1.183, 22.7078) ccw
  line L1908 (1.3238, 22.2161) -> (1.6661, 21.8738)
  arc A1910 (1.6661, 21.8738) -> (1.7551, 21.9628) centre (1.7106, 21.9183) ccw
  line L1909 (1.7551, 21.9628) -> (1.4128, 22.3051)
  arc A1911 (1.4128, 22.3051) -> (1.3238, 22.2161) centre (1.3683, 22.2606) ccw
  line L1910 (1.6865, 21.8601) -> (2.1337, 21.6748)
  arc A1912 (2.1337, 21.6748) -> (2.1819, 21.7912) centre (2.1578, 21.733) ccw
  line L1911 (2.1819, 21.7912) -> (1.7347, 21.9765)
  arc A1913 (1.7347, 21.9765) -> (1.6865, 21.8601) centre (1.7106, 21.9183) ccw
  line L1912 (3.5783, 33.2281) -> (3.5783, 33.6718)
  arc A1914 (3.5783, 33.6718) -> (3.4523, 33.6718) centre (3.5153, 33.6718) ccw
  line L1913 (3.4523, 33.6718) -> (3.4523, 33.2281)
  arc A1915 (3.4523, 33.2281) -> (3.5783, 33.2281) centre (3.5153, 33.2281) ccw
  line L1914 (3.5735, 33.6959) -> (3.4037, 34.1059)
  arc A1916 (3.4037, 34.1059) -> (3.2873, 34.0577) centre (3.3455, 34.0818) ccw
  line L1915 (3.2873, 34.0577) -> (3.4571, 33.6477)
  arc A1917 (3.4571, 33.6477) -> (3.5735, 33.6959) centre (3.5153, 33.6718) ccw
  line L1916 (3.39, 34.1263) -> (3.0763, 34.44)
  arc A1918 (3.0763, 34.44) -> (2.9873, 34.351) centre (3.0318, 34.3955) ccw
  line L1917 (2.9873, 34.351) -> (3.301, 34.0373)
  arc A1919 (3.301, 34.0373) -> (3.39, 34.1263) centre (3.3455, 34.0818) ccw
  line L1918 (3.0559, 34.4537) -> (2.6459, 34.6235)
  arc A1920 (2.6459, 34.6235) -> (2.5977, 34.5071) centre (2.6218, 34.5653) ccw
  line L1919 (2.5977, 34.5071) -> (3.0077, 34.3373)
  arc A1921 (3.0077, 34.3373) -> (3.0559, 34.4537) centre (3.0318, 34.3955) ccw
  line L1920 (2.6218, 34.6283) -> (2.1781, 34.6283)
  arc A1922 (2.1781, 34.6283) -> (2.1781, 34.5023) centre (2.1781, 34.5653) ccw
  line L1921 (2.1781, 34.5023) -> (2.6218, 34.5023)
  arc A1923 (2.6218, 34.5023) -> (2.6218, 34.6283) centre (2.6218, 34.5653) ccw
  line L1922 (2.154, 34.6235) -> (1.744, 34.4537)
  arc A1924 (1.744, 34.4537) -> (1.7922, 34.3373) centre (1.7681, 34.3955) ccw
  line L1923 (1.7922, 34.3373) -> (2.2022, 34.5071)
  arc A1925 (2.2022, 34.5071) -> (2.154, 34.6235) centre (2.1781, 34.5653) ccw
  line L1924 (1.7236, 34.44) -> (1.4099, 34.1263)
  arc A1926 (1.4099, 34.1263) -> (1.4989, 34.0373) centre (1.4544, 34.0818) ccw
  line L1925 (1.4989, 34.0373) -> (1.8126, 34.351)
  arc A1927 (1.8126, 34.351) -> (1.7236, 34.44) centre (1.7681, 34.3955) ccw
  line L1926 (1.3962, 34.1059) -> (1.2264, 33.6959)
  arc A1928 (1.2264, 33.6959) -> (1.3428, 33.6477) centre (1.2846, 33.6718) ccw
  line L1927 (1.3428, 33.6477) -> (1.5126, 34.0577)
  arc A1929 (1.5126, 34.0577) -> (1.3962, 34.1059) centre (1.4544, 34.0818) ccw
  line L1928 (1.2216, 33.6718) -> (1.2216, 33.2281)
  arc A1930 (1.2216, 33.2281) -> (1.3476, 33.2281) centre (1.2846, 33.2281) ccw
  line L1929 (1.3476, 33.2281) -> (1.3476, 33.6718)
  arc A1931 (1.3476, 33.6718) -> (1.2216, 33.6718) centre (1.2846, 33.6718) ccw
  line L1930 (1.2264, 33.204) -> (1.3962, 32.794)
  arc A1932 (1.3962, 32.794) -> (1.5126, 32.8422) centre (1.4544, 32.8181) ccw
  line L1931 (1.5126, 32.8422) -> (1.3428, 33.2522)
  arc A1933 (1.3428, 33.2522) -> (1.2264, 33.204) centre (1.2846, 33.2281) ccw
  line L1932 (1.4099, 32.7736) -> (1.7236, 32.4599)
  arc A1934 (1.7236, 32.4599) -> (1.8126, 32.5489) centre (1.7681, 32.5044) ccw
  line L1933 (1.8126, 32.5489) -> (1.4989, 32.8626)
  arc A1935 (1.4989, 32.8626) -> (1.4099, 32.7736) centre (1.4544, 32.8181) ccw
  line L1934 (1.744, 32.4462) -> (2.154, 32.2764)
  arc A1936 (2.154, 32.2764) -> (2.2022, 32.3928) centre (2.1781, 32.3346) ccw
  line L1935 (2.2022, 32.3928) -> (1.7922, 32.5626)
  arc A1937 (1.7922, 32.5626) -> (1.744, 32.4462) centre (1.7681, 32.5044) ccw
  line L1936 (2.1781, 32.2716) -> (2.6218, 32.2716)
  arc A1938 (2.6218, 32.2716) -> (2.6218, 32.3976) centre (2.6218, 32.3346) ccw
  line L1937 (2.6218, 32.3976) -> (2.1781, 32.3976)
  arc A1939 (2.1781, 32.3976) -> (2.1781, 32.2716) centre (2.1781, 32.3346) ccw
  line L1938 (2.6459, 32.2764) -> (3.0559, 32.4462)
  arc A1940 (3.0559, 32.4462) -> (3.0077, 32.5626) centre (3.0318, 32.5044) ccw
  line L1939 (3.0077, 32.5626) -> (2.5977, 32.3928)
  arc A1941 (2.5977, 32.3928) -> (2.6459, 32.2764) centre (2.6218, 32.3346) ccw
  line L1940 (3.0763, 32.4599) -> (3.39, 32.7736)
  arc A1942 (3.39, 32.7736) -> (3.301, 32.8626) centre (3.3455, 32.8181) ccw
  line L1941 (3.301, 32.8626) -> (2.9873, 32.5489)
  arc A1943 (2.9873, 32.5489) -> (3.0763, 32.4599) centre (3.0318, 32.5044) ccw
  line L1942 (3.4037, 32.794) -> (3.5735, 33.204)
  arc A1944 (3.5735, 33.204) -> (3.4571, 33.2522) centre (3.5153, 33.2281) ccw
  line L1943 (3.4571, 33.2522) -> (3.2873, 32.8422)
  arc A1945 (3.2873, 32.8422) -> (3.4037, 32.794) centre (3.3455, 32.8181) ccw
  line L1944 (2.1578, 35.67) -> (2.337, 35.67)
  arc A1946 (2.337, 35.67) -> (2.337, 35.796) centre (2.337, 35.733) ccw
  line L1945 (2.337, 35.796) -> (2.1578, 35.796)
  arc A1947 (2.1578, 35.796) -> (2.1578, 35.67) centre (2.1578, 35.733) ccw
  line L1946 (2.4, 35.733) -> (2.4, 36.8865)
  arc A1948 (2.4, 36.8865) -> (2.274, 36.8865) centre (2.337, 36.8865) ccw
  line L1947 (2.274, 36.8865) -> (2.274, 35.733)
  arc A1949 (2.274, 35.733) -> (2.4, 35.733) centre (2.337, 35.733) ccw
  line L1948 (2.337, 36.8235) -> (2.4628, 36.8235)
  arc A1950 (2.4628, 36.8235) -> (2.4628, 36.9495) centre (2.4628, 36.8865) ccw
  line L1949 (2.4628, 36.9495) -> (2.337, 36.9495)
  arc A1951 (2.337, 36.9495) -> (2.337, 36.8235) centre (2.337, 36.8865) ccw
  line L1950 (2.3998, 36.8865) -> (2.3998, 35.733)
  arc A1952 (2.3998, 35.733) -> (2.5258, 35.733) centre (2.4628, 35.733) ccw
  line L1951 (2.5258, 35.733) -> (2.5258, 36.8865)
  arc A1953 (2.5258, 36.8865) -> (2.3998, 36.8865) centre (2.4628, 36.8865) ccw
  line L1952 (2.4628, 35.67) -> (2.6421, 35.67)
  arc A1954 (2.6421, 35.67) -> (2.6421, 35.796) centre (2.6421, 35.733) ccw
  line L1953 (2.6421, 35.796) -> (2.4628, 35.796)
  arc A1955 (2.4628, 35.796) -> (2.4628, 35.67) centre (2.4628, 35.733) ccw
  line L1954 (2.6662, 35.6748) -> (3.1134, 35.8601)
  arc A1956 (3.1134, 35.8601) -> (3.0652, 35.9765) centre (3.0893, 35.9183) ccw
  line L1955 (3.0652, 35.9765) -> (2.618, 35.7912)
  arc A1957 (2.618, 35.7912) -> (2.6662, 35.6748) centre (2.6421, 35.733) ccw
  line L1956 (3.1338, 35.8738) -> (3.4761, 36.2161)
  arc A1958 (3.4761, 36.2161) -> (3.3871, 36.3051) centre (3.4316, 36.2606) ccw
  line L1957 (3.3871, 36.3051) -> (3.0448, 35.9628)
  arc A1959 (3.0448, 35.9628) -> (3.1338, 35.8738) centre (3.0893, 35.9183) ccw
  line L1958 (3.4898, 36.2365) -> (3.6751, 36.6837)
  arc A1960 (3.6751, 36.6837) -> (3.5587, 36.7319) centre (3.6169, 36.7078) ccw
  line L1959 (3.5587, 36.7319) -> (3.3734, 36.2847)
  arc A1961 (3.3734, 36.2847) -> (3.4898, 36.2365) centre (3.4316, 36.2606) ccw
  line L1960 (3.6799, 36.7078) -> (3.6799, 36.887)
  arc A1962 (3.6799, 36.887) -> (3.5539, 36.887) centre (3.6169, 36.887) ccw
  line L1961 (3.5539, 36.887) -> (3.5539, 36.7078)
  arc A1963 (3.5539, 36.7078) -> (3.6799, 36.7078) centre (3.6169, 36.7078) ccw
  line L1962 (3.6169, 36.95) -> (2.4634, 36.95)
  arc A1964 (2.4634, 36.95) -> (2.4634, 36.824) centre (2.4634, 36.887) ccw
  line L1963 (2.4634, 36.824) -> (3.6169, 36.824)
  arc A1965 (3.6169, 36.824) -> (3.6169, 36.95) centre (3.6169, 36.887) ccw
  line L1964 (2.5264, 36.887) -> (2.5264, 37.0128)
  arc A1966 (2.5264, 37.0128) -> (2.4004, 37.0128) centre (2.4634, 37.0128) ccw
  line L1965 (2.4004, 37.0128) -> (2.4004, 36.887)
  arc A1967 (2.4004, 36.887) -> (2.5264, 36.887) centre (2.4634, 36.887) ccw
  line L1966 (2.4634, 36.9498) -> (3.6169, 36.9498)
  arc A1968 (3.6169, 36.9498) -> (3.6169, 37.0758) centre (3.6169, 37.0128) ccw